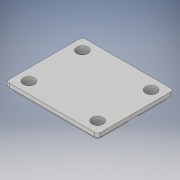
# Autodesk Inventor part: Enclosure_Top V3
Saved by Autodesk Inventor 2017 (Build 210142000, 142)
## iProperties
Created: 2017-12-18
Part Number: Enclosure_Top V3
Material: Generic
Document SubType Name: Modeling
Designer: Tripl_000
Density: 1 g/cm^3
Appearance: Default
Author: Tripl_000
Autodesk Inventor part; units mm, degrees
ref_plane "YZ Plane" through (0, 0, 0) normal (1, 0, 0) x (0, 1, 0)
ref_plane "XZ Plane" through (0, 0, 0) normal (0, 1, 0) x (-1, 0, 0)
ref_plane "XY Plane" through (0, 0, 0) normal (0, 0, 1) x (1, 0, 0)
sketch "Sketch1" plane through (0, 0, 0) normal (0, 1, 0) x (-1, 0, 0)
  line L0 (28, 23) -> (-28, 23)
  line L1 (-28, 23) -> (-28, -23)
  line L2 (-28, -23) -> (28, -23)
  line L3 (28, -23) -> (28, 23)
  line L4 (28, 23) -> (-28, -23) construction
  line L5 (-28, 23) -> (28, -23) construction
  point P0 (0, 0)
  dimension "d0" = 56
  dimension "d1" = 46
  constraints: 12 end point, 2 midpoint, 2 parallel, 1 horizontal, 1 perpendicular
  measures "d0" distance of L0.start L0.end
  measures "d1" distance of L2.end L0.start
extrude "Extrusion1" add sketch "Sketch1" along normal blind 2.5
sketch "Sketch2" plane through (0, 2.5, 0) normal (0, 1, 0) x (1, 0, 0)
  line L0 (-30, -25) -> (30, -25)
  line L1 (30, -25) -> (30, 25)
  line L2 (30, 25) -> (-30, 25)
  line L3 (-30, 25) -> (-30, -25)
  line L4 (-30, -25) -> (30, 25) construction
  line L5 (30, -25) -> (-30, 25) construction
  point P0 (0, 0)
  dimension "d4" = 50
  dimension "d5" = 60
  constraints: 12 end point, 2 midpoint, 2 parallel, 1 horizontal, 1 perpendicular
  measures "d4" distance of L2.end L0.start
  measures "d5" distance of L0.start L0.end
extrude "Extrusion2" add sketch "Sketch2" along normal blind 2.5
sketch "Sketch3" plane through (28, 0, 23) normal (1, 0, 0) x (0, 0, -1)
  line L0 (19.5, -2.5) -> (26.5, -2.5)
  line L1 (26.5, -2.5) -> (26.5, 2.5)
  line L2 (26.5, 2.5) -> (19.5, 2.5)
  line L3 (19.5, 2.5) -> (19.5, -2.5)
  line L4 (19.5, -2.5) -> (26.5, 2.5) construction
  line L5 (26.5, -2.5) -> (19.5, 2.5) construction
  point P0 (23, 0)
  dimension "d8" = 7
  dimension "d9" = 5
  constraints: 12 end point, 2 midpoint, 2 parallel, 1 horizontal, 1 perpendicular
  measures "d8" distance of L1.end L2.end
  measures "d9" distance of L0.end L1.end
extrude "Extrusion3" cut sketch "Sketch3" against normal through all
sketch "Sketch4" plane through (0, 5, 0) normal (0, 1, 0) x (1, 0, 0)
  line L0 (0, 31.16) -> (0, -35.6529)
  line L1 (-50.8705, 0) -> (45.6531, 0)
  circle A0 centre (-22.5, 17.5) radius 3.683
  circle A1 centre (22.5, 17.5) radius 3.683
  circle A2 centre (-22.5, -17.5) radius 3.683
  circle A3 centre (22.5, -17.5) radius 3.683
  point P0 (0, 0)
  dimension "d12" = 22.5
  dimension "d13" = 17.5
  dimension "d14" = 7.366
  constraints: 4 centre point, 4 end point, 3 symmetric about line, 1 horizontal, 1 vertical, 3 other
  measures "d12" horizontal distance of point (0, 0) A0.centre
  measures "d13" vertical distance of point (0, 0) A0.centre
  measures "d14" diameter of A0
fillet "Fillet1" radius 2 8 edges at (-28, 1.25, 23) (28, 1.25, 23) (28, 1.25, -23) (-28, 1.25, -23) (-30, 3.75, -25) (-30, 3.75, 25) (30, 3.75, 25) (30, 3.75, -25)
extrude "Extrusion5" cut sketch "Sketch4" against normal through all
body "Solid1"
